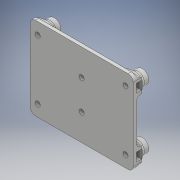
# Autodesk Inventor part: power
Saved by Autodesk Inventor 2018 (Build 220112000, 112)
## iProperties
Created: 2018-05-14
Part Number: power
Material: Generic
Document SubType Name: Modeling
Designer: bitbots
Density: 1 g/cm^3
Appearance: Default
Author: bitbots
Autodesk Inventor part; units mm, degrees
ref_plane "YZ Plane" through (0, 0, 0) normal (1, 0, 0) x (0, 1, 0)
ref_plane "XZ Plane" through (0, 0, 0) normal (0, 1, 0) x (-1, 0, 0)
ref_plane "XY Plane" through (0, 0, 0) normal (0, 0, 1) x (1, 0, 0)
sketch "Sketch1" plane through (0, 0, 0) normal (0, 1, 0) x (-1, 0, 0)
  line L0 (-31, 25) -> (31, 25)
  line L1 (31, 25) -> (31, -25)
  line L2 (31, -25) -> (-31, -25)
  line L3 (-31, -25) -> (-31, 25)
  line L4 (-31, 25) -> (31, -25) construction
  line L5 (31, 25) -> (-31, -25) construction
  point P0 (0, 0)
  dimension "d0" = 62
  dimension "d1" = 50
  constraints: 12 end point, 2 midpoint, 2 parallel, 1 horizontal, 1 perpendicular
  measures "d0" distance of L1.end L2.end
  measures "d1" distance of L0.end L1.end
extrude "Extrusion1" add sketch "Sketch1" along normal blind 2
sketch "Sketch2" plane through (0, 2, 0) normal (0, 1, 0) x (1, 0, 0)
  line L0 (26.5, -18) -> (-26.5, -18) construction
  line L1 (-26.5, -18) -> (-26.5, 18) construction
  line L2 (-26.5, 18) -> (26.5, 18) construction
  line L3 (26.5, 18) -> (26.5, -18) construction
  line L4 (26.5, -18) -> (-26.5, 18) construction
  line L5 (-26.5, -18) -> (26.5, 18) construction
  circle A0 centre (-26.5, -18) radius 4
  circle A1 centre (-26.5, 18) radius 4
  circle A2 centre (26.5, 18) radius 4
  circle A3 centre (26.5, -18) radius 4
  line L6 (-26.5, 18) -> (-26.5, 15.4)
  line L7 (22, 22.5) -> (31, 22.5)
  line L8 (31, 22.5) -> (31, 13.5)
  line L9 (31, 13.5) -> (22, 13.5)
  line L10 (22, 13.5) -> (22, 22.5)
  line L11 (22, 22.5) -> (31, 13.5) construction
  line L12 (31, 22.5) -> (22, 13.5) construction
  line L13 (22, -13.5) -> (31, -13.5)
  line L14 (31, -13.5) -> (31, -22.5)
  line L15 (31, -22.5) -> (22, -22.5)
  line L16 (22, -22.5) -> (22, -13.5)
  line L17 (22, -13.5) -> (31, -22.5) construction
  line L18 (31, -13.5) -> (22, -22.5) construction
  line L19 (-31, 22.5) -> (-22, 22.5)
  line L20 (-22, 22.5) -> (-22, 13.5)
  line L21 (-22, 13.5) -> (-31, 13.5)
  line L22 (-31, 13.5) -> (-31, 22.5)
  line L23 (-31, 22.5) -> (-22, 13.5) construction
  line L24 (-22, 22.5) -> (-31, 13.5) construction
  point P0 (0, 0)
  dimension "d4" = 53
  dimension "d5" = 36
  dimension "d6" = 8
  dimension "d7" = 8
  dimension "d8" = 8
  dimension "d9" = 8
  dimension "d32" = 2.6
  dimension "d37" = 9
  dimension "d38" = 9
  dimension "d39" = 9
  dimension "d40" = 9
  dimension "d41" = 9
  dimension "d42" = 9
  constraints: 50 end point, 8 midpoint, 8 parallel, 4 centre point, 4 coincident, 4 horizontal, 4 perpendicular, 1 point on line
  measures "d4" distance of L1.end L2.end
  measures "d5" distance of L0.end L1.end
  measures "d6" diameter of A0
  measures "d7" diameter of A1
  measures "d8" diameter of A2
  measures "d9" diameter of A3
  measures "d32" distance of L6.start L6.end
  measures "d37" distance of L8.end L9.end
  measures "d38" distance of L7.end L8.end
  measures "d39" distance of L14.end L15.end
  measures "d40" distance of L13.end L14.end
  measures "d41" distance of L20.end L21.end
  measures "d42" distance of L19.end L20.end
extrude "Extrusion2" add sketch "Sketch2" along normal blind 8 contours A0 | A1 | A2 | A3
sketch "Sketch3" plane through (-26.5, 10, 18) normal (0, 1, 0) x (1, 0, 0)
  circle A0 centre (0, 0) radius 4 projected
  circle A1 centre (0, 36) radius 4 projected
  circle A2 centre (53, 0) radius 4 projected
  circle A3 centre (53, 36) radius 4 projected
  circle A4 centre (0, 0) radius 1.5
  circle A5 centre (0, 36) radius 1.5
  circle A6 centre (53, 0) radius 1.5
  circle A7 centre (53, 36) radius 1.5
  point P0 (26.5, 18)
  dimension "d12" = 3
  dimension "d13" = 3
  dimension "d14" = 3
  dimension "d15" = 3
  constraints: 4 centre point, 4 coincident
  measures "d12" diameter of A4
  measures "d13" diameter of A5
  measures "d14" diameter of A6
  measures "d15" diameter of A7
extrude "Extrusion3" cut sketch "Sketch3" against normal through all contours A4 | A5 | A6 | A7
sketch "Sketch7" plane through (0, 2, 0) normal (0, 1, 0) x (1, 0, 0)
  circle A0 centre (26.5, 18) radius 1.5 projected
  circle A1 centre (26.5, 18) radius 4 projected
  line L0 (31, 22.5) -> (22, 22.5)
  line L1 (22, 22.5) -> (22, 13.5)
  line L2 (22, 13.5) -> (31, 13.5)
  line L3 (31, 13.5) -> (31, 22.5)
  circle A2 centre (26.5, 18) radius 1.5 projected
  line L4 (31, 22.5) -> (22, 13.5) construction
  line L5 (22, 22.5) -> (31, 13.5) construction
  point P0 (0, 0)
  dimension "d43" = 9
  dimension "d44" = 9
  constraints: 12 end point, 2 midpoint, 2 parallel, 1 horizontal, 1 perpendicular
  measures "d43" distance of L2.end L1.end
  measures "d44" distance of L1.end L0.end
extrude "Extrusion7" add sketch "Sketch7" along normal blind 3 contours L3 L2 L1 L0
mirror "Mirror3" about plane through (0, 0, 0) normal (0, 0, 1) of "Extrusion7"
mirror "Mirror4" about plane through (0, 0, 0) normal (1, 0, 0) of "Mirror3", "Extrusion7"
fillet "Fillet2" radius 2.36 16 edges at (22.5, 5, 18) (-30.5, 5, 18) (-30.5, 5, -18) (22.5, 5, -18) (26.5, 2, -22.5) (22, 2, -18) (26.5, 2, -13.5) (-26.5, 2, -13.5) (-26.5, 2, 13.5) (-26.5, 2, -22.5) (-22, 2, -18) (-22, 2, 18) (-26.5, 2, 22.5) (26.5, 2, 22.5) (22, 2, 18) (26.5, 2, 13.5)
sketch "Sketch4" plane through (0, 0, 0) normal (0, -1, 0) x (1, 0, 0)
  circle A0 centre (26.5, 18) radius 1.5 projected
  circle A1 centre (-26.5, 18) radius 1.5 projected
  circle A2 centre (-26.5, -18) radius 1.5 projected
  circle A3 centre (26.5, -18) radius 1.5 projected
  line L0 (31, 25) -> (-31, 25) projected
  line L1 (-31, 25) -> (-31, -25) projected
  line L2 (-31, -25) -> (31, -25) projected
  line L3 (31, -25) -> (31, 25) projected
  line L4 (31, 0) -> (1, 0)
  line L5 (0, 0) -> (0, -9)
  line L6 (0, 0) -> (0, 9)
  circle A4 centre (0, 9) radius 1.5
  circle A5 centre (0, -9) radius 1.5
  dimension "d20" = 9
  dimension "d21" = 9
  dimension "d22" = 3
  dimension "d23" = 3
  constraints: 6 end point, 2 centre point, 2 coincident, 2 vertical, 1 horizontal, 1 midpoint
  measures "d20" distance of L5.start L5.end
  measures "d21" distance of L5.start L6.end
  measures "d22" diameter of A4
  measures "d23" diameter of A5
extrude "Extrusion4" cut sketch "Sketch4" against normal through all contours A4 | A5
sketch "Sketch5" plane through (0, 2, 0) normal (0, 1, 0) x (1, 0, 0)
  circle A0 centre (0, 9) radius 1.5 projected
  circle A1 centre (0, -9) radius 1.5 projected
  line L0 (0, 9) -> (0, 11.6)
  line L1 (0, -9) -> (0, -11.6)
  line L2 (1.5011, 11.6) -> (3.0022, 9)
  line L3 (3.0022, 9) -> (1.5011, 6.4)
  line L4 (1.5011, 6.4) -> (-1.5011, 6.4)
  line L5 (-1.5011, 6.4) -> (-3.0022, 9)
  line L6 (-3.0022, 9) -> (-1.5011, 11.6)
  line L7 (-1.5011, 11.6) -> (1.5011, 11.6)
  line L8 (-1.5011, -11.6) -> (-3.0022, -9)
  line L9 (-3.0022, -9) -> (-1.5011, -6.4)
  line L10 (-1.5011, -6.4) -> (1.5011, -6.4)
  line L11 (1.5011, -6.4) -> (3.0022, -9)
  line L12 (3.0022, -9) -> (1.5011, -11.6)
  line L13 (1.5011, -11.6) -> (-1.5011, -11.6)
  line L14 (0, 11.6) -> (0, 13.6)
  line L15 (0, -11.6) -> (0, -13.6)
  line L16 (2.6558, 13.6) -> (5.3116, 9)
  line L17 (5.3116, 9) -> (2.6558, 4.4)
  line L18 (2.6558, 4.4) -> (-2.6558, 4.4)
  line L19 (-2.6558, 4.4) -> (-5.3116, 9)
  line L20 (-5.3116, 9) -> (-2.6558, 13.6)
  line L21 (-2.6558, 13.6) -> (2.6558, 13.6)
  line L22 (-2.6558, -13.6) -> (-5.3116, -9)
  line L23 (-5.3116, -9) -> (-2.6558, -4.4)
  line L24 (-2.6558, -4.4) -> (2.6558, -4.4)
  line L25 (2.6558, -4.4) -> (5.3116, -9)
  line L26 (5.3116, -9) -> (2.6558, -13.6)
  line L27 (2.6558, -13.6) -> (-2.6558, -13.6)
  point P0 (0, 0)
  dimension "d26" = 2.6
  dimension "d27" = 2.6
  dimension "d28" = 2
  dimension "d29" = 2
  constraints: 56 end point, 4 coincident, 4 midpoint, 4 vertical, 52 other
  measures "d26" distance of L0.start L0.end
  measures "d27" distance of L1.start L1.end
  measures "d28" distance of L0.end L14.end
  measures "d29" distance of L1.end L15.end
extrude "Extrusion5" add sketch "Sketch5" along normal blind 3 contours L16 L17 L18 L19 L20 L21 | L22 L23 L24 L25 L26 L27
sketch "Sketch6" plane through (0, 2, 0) normal (0, 1, 0) x (1, 0, 0)
  circle A0 centre (-26.5, 18) radius 1.5 projected
  circle A1 centre (26.5, 18) radius 1.5 projected
  circle A2 centre (26.5, -18) radius 1.5 projected
  circle A3 centre (-26.5, -18) radius 1.5 projected
  line L0 (-26.5, 18) -> (-26.5, 20.6)
  line L1 (-24.9989, 20.6) -> (-23.4978, 18)
  line L2 (-23.4978, 18) -> (-24.9989, 15.4)
  line L3 (-24.9989, 15.4) -> (-28.0011, 15.4)
  line L4 (-28.0011, 15.4) -> (-29.5022, 18)
  line L5 (-29.5022, 18) -> (-28.0011, 20.6)
  line L6 (-28.0011, 20.6) -> (-24.9989, 20.6)
  line L7 (-28.0011, 20.6) -> (-28.0011, 15.4)
  line L8 (-28.0011, 15.4) -> (-38.0011, 15.4)
  line L9 (-38.0011, 15.4) -> (-38.0011, 20.6)
  line L10 (-38.0011, 20.6) -> (-28.0011, 20.6)
  line L11 (-28.0011, 20.6) -> (-28.0011, 15.4)
  line L12 (-28.0011, 15.4) -> (-26.5, 15.4)
  line L13 (-26.5, 15.4) -> (-26.5, 20.6)
  line L14 (-26.5, 20.6) -> (-28.0011, 20.6)
  point P0 (0, 0)
  dimension "d33" = 2.6
  dimension "d34" = 10
  constraints: 30 end point, 5 equal length, 2 perpendicular, 2 vertical, 1 coincident, 1 midpoint, 13 other
  measures "d33" distance of L0.start L0.end
  measures "d34" distance of L3.end L8.end
extrude "Extrusion6" cut sketch "Sketch6" along normal blind 3 contours A0 L0 L6 L1 L2 L3 L13 | L0 L13 A0 | A0 L7 L6 L0 | L13 L3 L7 A0 | L7 L4 L5 | L5 L4 L8 L9 L10 picked at (-27.4875, 18.1113)
mirror "Mirror1" about plane through (0, 0, 0) normal (0, 0, 1) of "Extrusion6"
mirror "Mirror2" about plane through (0, 0, 0) normal (1, 0, 0) of "Extrusion6", "Mirror1"
fillet "Fillet3" radius 3 12 edges at (-3.9837, 2, -11.3) (0, 2, -13.6) (3.9837, 2, -11.3) (3.9837, 2, -6.7) (0, 2, -4.4) (-3.9837, 2, -6.7) (-3.9837, 2, 6.7) (-3.9837, 2, 11.3) (0, 2, 13.6) (3.9837, 2, 11.3) (3.9837, 2, 6.7) (0, 2, 4.4)
fillet "Fillet5" radius 3 4 edges at (-31, 1, 25) (-31, 1, -25) (31, 1, -25) (31, 1, 25)
body "Solid1"
